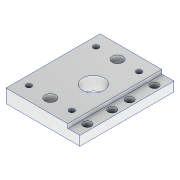
# Autodesk Inventor part: Techo, Vínculo Cabezal
Saved by Autodesk Inventor 2020 (Build 240168000, 168)
## iProperties
Created: 2020-05-11
Part Number: Techo, Vínculo Cabezal
Material: Aluminum 6061
Document SubType Name: Modeling
Designer: Dante
Density: 2.7 g/cm^3
Appearance: Aluminum - Flat
Mass: 84.2235 g
Surface Area: 112.016 cm^2
Volume: 31.1939 cm^3
Author: Dante
Autodesk Inventor part; units mm, degrees
ref_plane "YZ Plane" through (0, 0, 0) normal (1, 0, 0) x (0, 1, 0)
ref_plane "XZ Plane" through (0, 0, 0) normal (0, 1, 0) x (-1, 0, 0)
ref_plane "XY Plane" through (0, 0, 0) normal (0, 0, 1) x (1, 0, 0)
sketch "Sketch1" plane through (0, 0, 0) normal (0, 0, 1) x (1, 0, 0)
  line L0 (6.6074, 9.0814) -> (61.6074, 9.0814)
  line L1 (61.6074, 9.0814) -> (61.6074, 16.0814)
  line L2 (52.6074, 19.0814) -> (6.6074, 19.0814)
  line L3 (6.6074, 19.0814) -> (6.6074, 9.0814)
  line L4 (52.6074, 16.0814) -> (52.6074, 19.0814)
  line L5 (52.6074, 16.0814) -> (61.6074, 16.0814)
  point P0 (0, 0)
  dimension "d0" = 55
  dimension "d1" = 7
  dimension "d6" = 9
  dimension "d7" = 3
  constraints: 12 end point, 3 perpendicular, 2 horizontal, 1 vertical
  measures "d0" distance of L0.start L0.end
  measures "d1" distance of L0.end L1.end
  measures "d6" distance from line of L4.start L1
  measures "d7" distance of L2.start L4.start
extrude "Extrusion1" add sketch "Sketch1" along normal blind 70
sketch "Sketch2" plane through (6.6074, 19.0814, 0) normal (0, 1, 0) x (1, 0, 0)
  circle A0 centre (23, -10) radius 4
  circle A1 centre (23, -60) radius 4
  line L0 (46, -70) -> (0, -70) projected
  line L1 (55, 0) -> (55, -70) projected
  line L2 (46, 0) -> (0, 0) projected
  circle A2 centre (30, -35) radius 8
  line L3 (55, 0) -> (55, -70) projected
  circle A3 centre (50.5, -60) radius 3
  line L4 (46, 0) -> (46, -70) projected
  line L5 (55, -70) -> (46, -70) projected
  circle A4 centre (50.5, -41.5) radius 3
  circle A5 centre (50.5, -10) radius 3
  circle A6 centre (50.5, -28.5) radius 3
  line L6 (55, 0) -> (46, 0) projected
  line L7 (30, -43) -> (12.7252, -43)
  line L8 (23, -56) -> (14.0477, -56)
  line L9 (9, -14) -> (9, -56)
  line L10 (9, -56) -> (51, -56)
  line L11 (51, -56) -> (51, -14)
  line L12 (51, -14) -> (9, -14)
  circle A7 centre (14.5, -19.5) radius 2
  circle A8 centre (45.5, -19.5) radius 2
  circle A9 centre (45.5, -50.5) radius 2
  circle A10 centre (14.5, -51.5) radius 2
  line L13 (1, -101.1728) -> (51, -101.1728)
  circle A11 centre (39, -60) radius 2
  circle A12 centre (7, -60) radius 2
  circle A13 centre (30, -35) radius 12.5
  circle A14 centre (7, -60) radius 4
  circle A15 centre (39, -60) radius 4
  line L14 (0, 0) -> (0, -70) projected
  line L15 (0, -35) -> (-6.6074, -35)
  circle A16 centre (39, -10) radius 2
  circle A17 centre (7, -10) radius 2
  circle A18 centre (7, -10) radius 4
  circle A19 centre (39, -10) radius 4
  line L16 (37, -60) -> (37, -51.6268)
  line L17 (35, -60) -> (35, -52.1291)
  circle A20 centre (23, -60) radius 9
  line L18 (11, -60) -> (11, -66.8543)
  line L19 (14, -60) -> (14, -67.7509)
  line L20 (32, -60) -> (32, -67.7509)
  circle A21 centre (23, -60) radius 10
  line L21 (13, -60) -> (13, -90.2082)
  circle A22 centre (7, -97.0024) radius 2
  line L22 (13, -90.2082) -> (13, -105.086)
  circle A23 centre (39, -97.0024) radius 2
  line L23 (51, -101.1728) -> (51, -88.3214)
  line L24 (33, -60) -> (33, -163.1603)
  line L25 (1, -101.1728) -> (1, -81.8849)
  circle A24 centre (50.5, -105.086) radius 6.5
  line L26 (43, -90.2082) -> (43, -98.586)
  point P0 (-6.6074, 0)
  dimension "d11" = 8
  dimension "d17" = 16
  dimension "d55" = 4
  dimension "d64" = 8
  dimension "d65" = 8
  dimension "d10" = 8
  dimension "d12" = 10
  dimension "d15" = 10
  dimension "d18" = 35
  dimension "d22" = 6
  dimension "d23" = 4.5
  dimension "d24" = 10
  dimension "d30" = 10
  dimension "d33" = 32
  dimension "d34" = 32
  dimension "d35" = 25
  dimension "d36" = 4.5
  dimension "d37" = 4.5
  dimension "d40" = 42
  dimension "d41" = 42
  dimension "d42" = 42
  dimension "d43" = 4
  dimension "d44" = 4
  dimension "d45" = 4
  dimension "d46" = 4
  dimension "d47" = 31
  dimension "d48" = 31
  dimension "d50" = 32
  dimension "d51" = 5.5
  dimension "d52" = 5.5
  dimension "d53" = 5.5
  dimension "d54" = 50
  dimension "d56" = 4
  dimension "d59" = 60
  dimension "d60" = 60
  dimension "d61" = 21
  dimension "d62" = 5.5
  dimension "d63" = 25
  dimension "d69" = 7
  dimension "d71" = 18
  dimension "d72" = 14
  dimension "d73" = 14
  dimension "d74" = 20
  dimension "d75" = 4
  dimension "d76" = 4
  dimension "d79" = 6
  dimension "d80" = 6
  dimension "d83" = 12
  dimension "d84" = 13
  dimension "d86" = 8
  dimension "d129" = 28.5
  dimension "d130" = 28.5
  constraints: 38 end point, 20 centre point, 11 vertical, 7 coincident, 4 point on circle, 4 symmetric about line, 3 horizontal, 3 horizontal alignment, 2 perpendicular, 2 vertical alignment, 1 midpoint, 14 other
  measures "d10" diameter of A0
  measures "d12" distance from line of point (23, -60) L0
  measures "d15" distance from line of L2 A0.centre
  measures "d18" distance from line of point (30, -35) L0
  measures "d22" diameter of A3
  measures "d23" distance from line of A3.centre L4
  measures "d24" distance from line of L5 A3.centre
  measures "d30" distance from line of L6 A5.centre
  measures "d33" distance from line of A0.centre L1
  measures "d34" distance from line of point (23, -60) L1
  measures "d35" distance from line of point (30, -35) L1
  measures "d36" distance from line of L1 A5.centre
  measures "d37" distance from line of A6.centre L3
  measures "d40" distance of L9.start L9.end
  measures "d41" distance of L9.end L10.end
  measures "d42" distance of L10.end L11.end
  measures "d43" diameter of A7
  measures "d44" diameter of A8
  measures "d45" diameter of A9
  measures "d46" diameter of A10
  measures "d47" distance of A7.centre A8.centre
  measures "d48" distance of A9.centre A8.centre
  measures "d50" distance of A10.centre A7.centre
  measures "d51" distance from line of L12 A8.centre
  measures "d52" distance from line of A7.centre L12
  measures "d53" distance from line of L11 A8.centre
  measures "d54" distance of L13.start L13.end
  measures "d56" diameter of A12
  measures "d59" distance from line of A12.centre L2
  measures "d60" distance from line of L2 point (39, -60)
  measures "d61" distance from line of L9 point (30, -35)
  measures "d62" distance from line of L11 A9.centre
  measures "d63" diameter of A13
  measures "d69" distance from line of point (39, -60) L4
  measures "d71" diameter of A20
  measures "d72" distance between parallel lines of L14 L19
  measures "d73" distance between parallel lines of L20 L4
  measures "d74" diameter of A21
  measures "d75" diameter of A22
  measures "d76" diameter of A23
  measures "d79" distance from line of L24 A23.centre
  measures "d80" distance from line of A22.centre L22
  measures "d83" distance between parallel lines of L25 L22
  measures "d84" diameter of A24
  measures "d86" distance between parallel lines of L26 L23
  measures "d129" distance from line of A6.centre L6
  measures "d130" distance from line of L5 A4.centre
extrude "Extrusion2" cut sketch "Sketch2" against normal blind 30 contours A0 | L11 A6 | A6 L11 | A1 | L11 A4 | A4 L11 | A2 | A3 | A5
sketch "Sketch4" plane through (6.6074, 9.0814, 0) normal (0, -1, 0) x (1, 0, 0)
  circle A0 centre (7, 60) radius 2
  circle A1 centre (39, 60) radius 2
  circle A2 centre (7, 10) radius 2
  circle A3 centre (39, 10) radius 2
  dimension "d97" = 4
  dimension "d98" = 4
  dimension "d99" = 4
  constraints: 4 centre point
  measures "d97" diameter of A0
  measures "d98" diameter of A2
  measures "d99" diameter of A3
extrude "Extrusion4" cut sketch "Sketch4" against normal blind 70
sketch "Boceto5" plane through (6.6074, 9.0814, 0) normal (-1, 0, 0) x (0, 0, 1)
  circle A0 centre (38.25, 7) radius 1
  circle A1 centre (31.75, 7) radius 1
  line L0 (70, 10) -> (70, 0) projected
  line L1 (0, 10) -> (70, 10) projected
  line L2 (35, 6.1177) -> (35, -0.846)
  point P0 (0, -9.0814)
  dimension "d106" = 2
  dimension "d139" = 3
  dimension "d140" = 2
  dimension "d141" = 3
  dimension "d142" = 6.5
  dimension "d143" = 3.25
  dimension "d144" = 35
  constraints: 2 centre point, 2 end point, 1 coincident, 1 vertical
  measures "d106" diameter of A1
  measures "d139" distance from line of L1 A0.centre
  measures "d140" diameter of A0
  measures "d141" distance from line of L1 point (31.75, 7)
  measures "d142" distance of point (31.75, 7) A0.centre
  measures "d143" distance from line of L2 A0.centre
  measures "d144" distance between parallel lines of L0 L2
hole "Agujero1" at (6.6074, 16.0814, 38.25) at (6.6074, 16.0814, 31.75) direction (1, 0, 0) diameter 2 depth 15 tip angle 120
thread "Thread3" size "M4x0.7" class "6H" standard "ISO Metric profile" length 98
thread "Thread4" size "M4x0.7" class "6H" standard "ISO Metric profile" length 98
thread "Thread5" size "M4x0.7" class "6H" standard "ISO Metric profile" length 98
thread "Thread6" size "M4x0.7" class "6H" standard "ISO Metric profile" length 98
thread "Thread7" size "M2x0.4" class "6H" standard "ISO Metric profile" length 12
thread "Thread8" size "M2x0.4" class "6H" standard "ISO Metric profile" length 12
body "Solid1"
